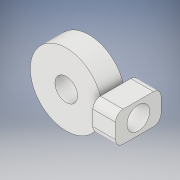
# Autodesk Inventor part: Arm7
Saved by Autodesk Inventor 2017 SP1 (Build 210196100, 196)
## iProperties
Created: 2018-02-11
Part Number: Arm7
Material: ABS Plastic
Document SubType Name: Modeling
Designer: Zach
Density: 1.06 g/cm^3
Appearance: CR White
Author: Zach
Autodesk Inventor part; units mm, degrees
ref_plane "YZ Plane" through (0, 0, 0) normal (1, 0, 0) x (0, 1, 0)
ref_plane "XZ Plane" through (0, 0, 0) normal (0, 1, 0) x (-1, 0, 0)
ref_plane "XY Plane" through (0, 0, 0) normal (0, 0, 1) x (1, 0, 0)
sketch "Sketch1" plane through (0, 0, 0) normal (0, 0, 1) x (1, 0, 0)
  circle A0 centre (0, 0) radius 1.5
  circle A1 centre (0, 0) radius 4.75
  dimension "d0" = 3
  dimension "d1" = 9.5
  constraints: 2 centre point, 2 coincident
  measures "d0" diameter of A0
  measures "d1" diameter of A1
extrude "Extrusion1" add sketch "Sketch1" along normal blind 3
sketch "Sketch2" plane through (0, 0, 3) normal (0, 0, 1) x (1, 0, 0)
  circle A0 centre (0, 0) radius 4.75 projected
  line L0 (4.5069, 1.5) -> (5.0069, 1.5)
  line L1 (5.0069, 1.5) -> (5.0069, -1.5)
  line L2 (5.0069, -1.5) -> (4.5069, -1.5)
  line L3 (4.5069, -1.5) -> (4.5069, 1.5)
  point P0 (4.5069, 0)
  dimension "d4" = 3
  dimension "d5" = 0.5
  constraints: 8 end point, 2 parallel, 2 point on circle, 1 horizontal, 1 midpoint, 1 perpendicular
  measures "d4" distance of L0.end L1.end
  measures "d5" distance of L0.start L0.end
extrude "Extrusion2" add sketch "Sketch2" against normal blind 3 contours A0 L0 L1 L2
sketch "Sketch4" plane through (5.0069, -1.5, 3) normal (1, 0, 0) x (0, 0, -1)
  line L0 (-1.5, 3.5) -> (4.5, 3.5)
  line L1 (4.5, 3.5) -> (4.5, -0.5)
  line L2 (4.5, -0.5) -> (-1.5, -0.5)
  line L3 (-1.5, -0.5) -> (-1.5, 3.5)
  line L4 (0, 3) -> (3, 3) projected
  line L5 (0, 0) -> (0, 3) projected
  point P0 (3, 1.5)
  point P1 (1.5, 3)
  point P2 (1.5, 3.5)
  point P3 (0, 1.5)
  point P4 (-1.5, 1.5)
  dimension "d9" = 6
  dimension "d10" = 4
  constraints: 8 end point, 4 midpoint, 2 parallel, 1 horizontal, 1 horizontal alignment, 1 perpendicular, 1 vertical alignment
  measures "d9" distance of L0.start L0.end
  measures "d10" distance of L0.end L1.end
extrude "Extrusion3" add sketch "Sketch4" along normal blind 3
fillet "Fillet1" radius 1 4 edges at (6.5069, 2, 4.5) (6.5069, -2, 4.5) (6.5069, -2, -1.5) (6.5069, 2, -1.5)
sketch "Sketch6" plane through (8.0069, -1.5, 3) normal (1, 0, 0) x (0, 0, -1)
  circle A0 centre (1.5, 1.5) radius 1.5
  line L0 (3.5, 3.5) -> (-0.5, 3.5) projected
  line L1 (-1.5, 2.5) -> (-1.5, 0.5) projected
  point P0 (3, 1.5)
  point P1 (-1.5, 1.5)
  point P2 (1.5, 3.5)
  dimension "d14" = 3
  constraints: 2 midpoint, 1 centre point, 1 horizontal alignment, 1 vertical alignment
  measures "d14" diameter of A0
extrude "Extrusion4" cut sketch "Sketch6" against normal blind 3
body "Solid1"
